Autodesk Fusion 360 part; units mm, degrees
(part 2 of 3)
  spline S100 degree 3 poles (29.5625, 4.9912) (29.775, 5.0168) (30.2128, 5.0697) (30.5239, 5.3836) (30.6839, 5.5451) knots 0 0 0 0 0.062335 0.128396 0.128396 0.128396 0.128396
  spline S101 degree 3 poles (30.6839, 5.5451) (30.8194, 5.7748) (31.1299, 6.3011) (31.1431, 6.9153) (31.1505, 7.2613) knots 0 0 0 0 0.078797 0.180491 0.180491 0.180491 0.180491
  spline S102 degree 3 poles (31.1505, 7.2613) (31.1422, 7.593) (31.1274, 8.1866) (30.8272, 8.6957) (30.6948, 8.9203) knots 0 0 0 0 0.09753 0.174557 0.174557 0.174557 0.174557
  spline S103 degree 3 poles (30.6948, 8.9203) (30.5395, 9.081) (30.2395, 9.3914) (29.8122, 9.4454) (29.6061, 9.4714) knots 0 0 0 0 0.064875 0.125334 0.125334 0.125334 0.125334
  spline S104 degree 3 poles (29.6061, 9.4714) (29.399, 9.442) (28.9607, 9.3797) (28.6562, 9.0557) (28.4956, 8.8848) knots 0 0 0 0 0.060932 0.128979 0.128979 0.128979 0.128979
  spline S105 degree 3 poles (28.4956, 8.8848) (28.3552, 8.6509) (28.0416, 8.1287) (28.023, 7.5171) (28.0127, 7.1795) knots 0 0 0 0 0.080566 0.17987 0.17987 0.17987 0.17987
  line L143 (35.4834, 5.1931) -> (35.6252, 4.3254)
  spline S106 degree 3 poles (35.6252, 4.3254) (35.4947, 4.3) (35.2494, 4.2522) (34.9998, 4.2426) (34.8831, 4.2381) knots 0 0 0 0 0.039832 0.074826 0.074826 0.074826 0.074826
  spline S107 degree 3 poles (34.8831, 4.2381) (34.7224, 4.2412) (34.4348, 4.2468) (34.1703, 4.3581) (34.0536, 4.4073) knots 0 0 0 0 0.047664 0.085336 0.085336 0.085336 0.085336
  spline S108 degree 3 poles (34.0536, 4.4073) (33.9634, 4.4665) (33.7887, 4.5812) (33.6877, 4.7638) (33.6389, 4.8521) knots 0 0 0 0 0.031834 0.061632 0.061632 0.061632 0.061632
  spline S109 degree 3 poles (33.6389, 4.8521) (33.6044, 4.9941) (33.512, 5.3741) (33.5162, 5.7661) (33.5188, 6.0117) knots 0 0 0 0 0.043707 0.116961 0.116961 0.116961 0.116961
  line L144 (33.5188, 6.0117) -> (33.5188, 9.3459)
  line L145 (33.5188, 9.3459) -> (32.7985, 9.3459)
  line L146 (32.7985, 9.3459) -> (32.7985, 10.1099)
  line L147 (32.7985, 10.1099) -> (33.5188, 10.1099)
  line L148 (33.5188, 10.1099) -> (33.5188, 11.5451)
  line L149 (33.5188, 11.5451) -> (34.4956, 12.1345)
  line L150 (34.4956, 12.1345) -> (34.4956, 10.1099)
  line L151 (34.4956, 10.1099) -> (35.4834, 10.1099)
  line L152 (35.4834, 10.1099) -> (35.4834, 9.3459)
  line L153 (35.4834, 9.3459) -> (34.4956, 9.3459)
  line L154 (34.4956, 9.3459) -> (34.4956, 5.9571)
  spline S110 degree 3 poles (34.4956, 5.9571) (34.4942, 5.8414) (34.4919, 5.659) (34.5326, 5.4817) (34.5475, 5.4169) knots 0 0 0 0 0.03454 0.054433 0.054433 0.054433 0.054433
  spline S111 degree 3 poles (34.5475, 5.4169) (34.5677, 5.3787) (34.6088, 5.3015) (34.6804, 5.2513) (34.7166, 5.2259) knots 0 0 0 0 0.012755 0.025838 0.025838 0.025838 0.025838
  spline S112 degree 3 poles (34.7166, 5.2259) (34.7635, 5.2052) (34.8701, 5.1584) (34.9868, 5.1562) (35.0522, 5.1549) knots 0 0 0 0 0.015217 0.034603 0.034603 0.034603 0.034603
  spline S113 degree 3 poles (35.0522, 5.1549) (35.1155, 5.1572) (35.2599, 5.1623) (35.403, 5.182) (35.4834, 5.1931) knots 0 0 0 0 0.018987 0.043304 0.043304 0.043304 0.043304
  line L155 (36.4001, 2.0826) -> (36.291, 3.0048)
  spline S114 degree 3 poles (36.291, 3.0048) (36.391, 2.9794) (36.5756, 2.9325) (36.7658, 2.9222) (36.8531, 2.9175) knots 0 0 0 0 0.030853 0.057001 0.057001 0.057001 0.057001
  spline S115 degree 3 poles (36.8531, 2.9175) (36.9528, 2.92) (37.1344, 2.9246) (37.3015, 2.9949) (37.3769, 3.0267) knots 0 0 0 0 0.029594 0.053932 0.053932 0.053932 0.053932
  spline S116 degree 3 poles (37.3769, 3.0267) (37.4397, 3.067) (37.5663, 3.1484) (37.6544, 3.2706) (37.6989, 3.3323) knots 0 0 0 0 0.022157 0.044743 0.044743 0.044743 0.044743
  spline S117 degree 3 poles (37.6989, 3.3323) (37.7407, 3.4172) (37.8571, 3.654) (37.9436, 3.9035) (37.999, 4.0635) knots 0 0 0 0 0.028377 0.079105 0.079105 0.079105 0.079105
  spline S118 degree 3 poles (37.999, 4.0635) (38.0107, 4.0972) (38.0387, 4.1777) (38.0688, 4.2573) (38.0864, 4.3036) knots 0 0 0 0 0.0107 0.02555 0.02555 0.02555 0.02555
  line L156 (38.0864, 4.3036) -> (35.8872, 10.1099)
  line L157 (35.8872, 10.1099) -> (36.9458, 10.1099)
  line L158 (36.9458, 10.1099) -> (38.1518, 6.7538)
  spline S119 degree 3 poles (38.1518, 6.7538) (38.2285, 6.5363) (38.3845, 6.0939) (38.5088, 5.6414) (38.572, 5.4114) knots 0 0 0 0 0.069157 0.140705 0.140705 0.140705 0.140705
  spline S120 degree 3 poles (38.572, 5.4114) (38.631, 5.6351) (38.7483, 6.0806) (38.9002, 6.5155) (38.9759, 6.732) knots 0 0 0 0 0.069376 0.138143 0.138143 0.138143 0.138143
  line L159 (38.9759, 6.732) -> (40.2146, 10.1099)
  line L160 (40.2146, 10.1099) -> (41.1969, 10.1099)
  line L161 (41.1969, 10.1099) -> (38.9922, 4.2163)
  spline S121 degree 3 poles (38.9922, 4.2163) (38.8921, 3.9454) (38.7272, 3.499) (38.5218, 3.0699) (38.4411, 2.9012) knots 0 0 0 0 0.086568 0.142661 0.142661 0.142661 0.142661
  spline S122 degree 3 poles (38.4411, 2.9012) (38.3557, 2.7537) (38.1975, 2.4803) (37.9533, 2.2809) (37.8408, 2.189) knots 0 0 0 0 0.050608 0.093822 0.093822 0.093822 0.093822
  spline S123 degree 3 poles (37.8408, 2.189) (37.7198, 2.123) (37.4683, 1.9857) (37.1818, 1.9705) (37.0332, 1.9626) knots 0 0 0 0 0.04081 0.084832 0.084832 0.084832 0.084832
  spline S124 degree 3 poles (37.0332, 1.9626) (36.9324, 1.9688) (36.7165, 1.9821) (36.5102, 2.0476) (36.4001, 2.0826) knots 0 0 0 0 0.030163 0.064648 0.064648 0.064648 0.064648
extrude "Extrude11'" cut sketch "Sketch9" against normal blind 0.1 contours L94 L95 L96 S34 S35 S36 S37 S38 S39 S40 S41 S42 S43 L97 L98 sketch seen with x (1, 0, 0) y (0, 0, -1) z (0, 1, 0) at (0, -23.4903, 46.4903) bodies 3 in component "Component"
extrude "Extrude12'" cut sketch "Sketch9" against normal blind 0.1 contours L76 L77 L78 L79 L80 L81 L82 L83 L84 L85 L86 L87 | L88 S0 S1 S2 S3 S4 S5 S6 S7 S8 L89 S9 S10 S11 S12 | L91 S17 S18 S19 S20 S21 S22 S23 S24 S25 L92 S26 S27 S28 S29 | L99 L100 L101 S52 S53 L102 L103 L104 L105 L106 L107 L108 L109 L110 L111 | L112 S54 S55 S56 S57 S58 S59 S60 S61 S62 L113 S63 S64 S65 S66 | L115 L116 L117 L118 L119 L120 L121 L122 L123 L124 L125 L126 | L127 L128 L129 S71 S72 S73 S74 S75 S76 S77 L130 L131 L132 S78 S79 S80 S81 S82 L133 L134 L135 S83 S84 S85 S86 S87 L136 L137 | L138 L139 L140 S88 S89 S90 S91 S92 S93 S94 S95 S96 S97 L141 L142 | L143 S106 S107 S108 S109 L144 L145 L146 L147 L148 L149 L150 L151 L152 L153 L154 S110 S111 S112 S113 | L155 S114 S115 S116 S117 S118 L156 L157 L158 S119 S120 L159 L160 L161 S121 S122 S123 S124 sketch seen with x (1, 0, 0) y (0, 0, -1) z (0, 1, 0) at (0, -23.4903, 46.4903) bodies 3 in component "Component"
sketch "Sketch10" plane through (0, 0, 22.6977) normal (0, 0, 1) x (1, 0, 0)
  line L0 (-6.4359, 98.3368) -> (-6.4359, 103.3368)
  line L1 (-6.4359, 103.3368) -> (-8.4359, 103.3368)
  line L2 (-8.4359, 103.3368) -> (-8.4359, 108.3368)
  line L3 (-8.4359, 108.3368) -> (-6.4359, 108.3368)
  line L4 (-6.4359, 108.3368) -> (-6.4359, 113.3368)
  line L5 (-6.4359, 113.3368) -> (-56.4359, 113.3368)
  line L6 (-56.4359, 113.3368) -> (-56.4359, 108.3368)
  line L7 (-56.4359, 108.3368) -> (-53.4359, 108.3368)
  line L8 (-53.4359, 108.3368) -> (-53.4359, 103.3368)
  line L9 (-53.4359, 103.3368) -> (-56.4359, 103.3368)
  line L10 (-56.4359, 103.3368) -> (-56.4359, 98.3368)
  line L11 (-56.4359, 98.3368) -> (-53.4359, 98.3368)
  line L12 (-53.4359, 98.3368) -> (-53.4359, 93.3368)
  line L13 (-53.4359, 93.3368) -> (-56.4359, 93.3368)
  line L14 (-56.4359, 93.3368) -> (-56.4359, 88.3368)
  line L15 (-56.4359, 88.3368) -> (-53.4359, 88.3368)
  line L16 (-53.4359, 88.3368) -> (-53.4359, 83.3368)
  line L17 (-53.4359, 83.3368) -> (-56.4359, 83.3368)
  line L18 (-56.4359, 83.3368) -> (-56.4359, 78.3368)
  line L19 (-56.4359, 78.3368) -> (-53.4359, 78.3368)
  line L20 (-53.4359, 78.3368) -> (-53.4359, 73.3368)
  line L21 (-53.4359, 73.3368) -> (-56.4359, 73.3368)
  line L22 (-56.4359, 73.3368) -> (-56.4359, 68.3368)
  line L23 (-56.4359, 68.3368) -> (-46.7359, 68.3368)
  line L24 (-46.7359, 68.3368) -> (-46.7359, 65.8368)
  line L25 (-46.7359, 65.8368) -> (-41.3359, 65.8368)
  line L26 (-41.3359, 65.8368) -> (-41.3359, 68.3368)
  line L27 (-41.3359, 68.3368) -> (-36.7359, 68.3368)
  line L28 (-36.7359, 68.3368) -> (-36.7359, 65.8368)
  line L29 (-36.7359, 65.8368) -> (-31.3359, 65.8368)
  line L30 (-31.3359, 65.8368) -> (-31.3359, 68.3368)
  line L31 (-31.3359, 68.3368) -> (-26.7359, 68.3368)
  line L32 (-26.7359, 68.3368) -> (-26.7359, 65.8368)
  line L33 (-26.7359, 65.8368) -> (-21.3359, 65.8368)
  line L34 (-21.3359, 65.8368) -> (-21.3359, 68.3368)
  line L35 (-21.3359, 68.3368) -> (-16.7359, 68.3368)
  line L36 (-16.7359, 68.3368) -> (-16.7359, 65.8368)
  line L37 (-16.7359, 65.8368) -> (-11.3359, 65.8368)
  line L38 (-11.3359, 65.8368) -> (-11.3359, 68.3368)
  line L39 (-11.3359, 68.3368) -> (-6.4359, 68.3368)
  line L40 (-6.4359, 68.3368) -> (-6.4359, 73.3368)
  line L41 (-6.4359, 73.3368) -> (-8.4359, 73.3368)
  line L42 (-8.4359, 73.3368) -> (-8.4359, 78.3368)
  line L43 (-8.4359, 78.3368) -> (-6.4359, 78.3368)
  line L44 (-6.4359, 78.3368) -> (-6.4359, 83.3368)
  line L45 (-6.4359, 83.3368) -> (-8.4359, 83.3368)
  line L46 (-8.4359, 83.3368) -> (-8.4359, 88.3368)
  line L47 (-8.4359, 88.3368) -> (-6.4359, 88.3368)
  line L48 (-6.4359, 88.3368) -> (-6.4359, 93.3368)
  line L49 (-6.4359, 93.3368) -> (-8.4359, 93.3368)
  line L50 (-8.4359, 93.3368) -> (-8.4359, 98.3368)
  line L51 (-8.4359, 98.3368) -> (-6.4359, 98.3368)
  line L52 (-44.847, 105.1125) -> (-15.0997, 105.1125)
  line L53 (-15.0997, 105.1125) -> (-15.0997, 75.3652)
  line L54 (-15.0997, 75.3652) -> (-44.847, 75.3652)
  line L55 (-44.847, 75.3652) -> (-44.847, 105.1125)
  line L56 (-44.847, 105.1125) -> (-15.0997, 105.1125)
  line L57 (-44.847, 75.3652) -> (-44.847, 105.1125)
  line L58 (-15.0997, 75.3652) -> (-44.847, 75.3652)
  line L59 (-15.0997, 105.1125) -> (-15.0997, 75.3652)
  line L60 (-29.9733, 105.1125) -> (-29.9733, 75.3652) construction
  line L61 (-44.847, 90.2388) -> (-15.0997, 90.2388) construction
  line L62 (-8.6718, 90.2601) -> (-29.7064, 69.2256)
  line L63 (-29.7064, 69.2256) -> (-50.7409, 90.2601)
  line L64 (-29.7064, 111.2947) -> (-8.6718, 90.2601)
  line L65 (-50.7409, 90.2601) -> (-29.7064, 111.2947)
  line L66 (-16.0997, 76.3652) -> (-43.847, 76.3652)
  line L67 (-43.847, 76.3652) -> (-43.847, 104.1125)
  line L68 (-43.847, 104.1125) -> (-16.0997, 104.1125)
  line L69 (-16.0997, 104.1125) -> (-16.0997, 76.3652)
  line L70 (-49.3267, 90.2601) -> (-29.7064, 109.8804)
  line L71 (-29.7064, 109.8804) -> (-10.086, 90.2601)
  line L72 (-10.086, 90.2601) -> (-29.7064, 70.6398)
  line L73 (-29.7064, 70.6398) -> (-49.3267, 90.2601)
  dimension "d133" = 1
  dimension "d134" = 1
  constraint horizontal L52
  constraint vertical L53
  constraint horizontal L54
  constraint vertical L55
  constraint horizontal L56
  constraint vertical L59
  constraint horizontal L58
  constraint vertical L57
  constraint midpoint L56 L60.start
  constraint midpoint L54 L60.end
  constraint perpendicular L54 L60
  constraint midpoint L57 L61.start
  constraint midpoint L59 L61.end
extrude "Extrude3''" cut sketch "Sketch10" against normal blind 3 contours L52 L56 L70 L71 | L65 L67 L68 | L55 L57 L70 L73 | L66 L67 L68 L69 L70 L71 L72 L73 | L64 L68 L69 | L63 L66 L67 | L53 L59 L71 L72 | L54 L58 L72 L73 | L62 L66 L69 sketch seen with x (0, 0, -1) y (0, 1, 0) z (1, 0, 0) at (-19.6977, -54.1484, -8.993) bodies 4 in component "Component''"
sketch "Sketch11" plane through (0, 0, 2.5) normal (0, 0, 1) x (1, 0, 0)
  line L0 (47.5, 60) -> (47.5, 67.3)
  line L1 (47.5, 67.3) -> (50, 67.3)
  line L2 (50, 67.3) -> (50, 72.7)
  line L3 (50, 72.7) -> (47.5, 72.7)
  line L4 (47.5, 72.7) -> (47.5, 77.3)
  line L5 (47.5, 77.3) -> (50, 77.3)
  line L6 (50, 77.3) -> (50, 82.7)
  line L7 (50, 82.7) -> (47.5, 82.7)
  line L8 (47.5, 82.7) -> (47.5, 87.3)
  line L9 (47.5, 87.3) -> (50, 87.3)
  line L10 (50, 87.3) -> (50, 92.7)
  line L11 (50, 92.7) -> (47.5, 92.7)
  line L12 (47.5, 92.7) -> (47.5, 97.3)
  line L13 (47.5, 97.3) -> (50, 97.3)
  line L14 (50, 97.3) -> (50, 102.7)
  line L15 (50, 102.7) -> (47.5, 102.7)
  line L16 (47.5, 102.7) -> (47.5, 107.5)
  line L17 (47.5, 107.5) -> (2.5, 107.5)
  line L18 (2.5, 107.5) -> (2.5, 102.7)
  line L19 (2.5, 102.7) -> (0, 102.7)
  line L20 (0, 102.7) -> (0, 97.3)
  line L21 (0, 97.3) -> (2.5, 97.3)
  line L22 (2.5, 97.3) -> (2.5, 92.7)
  line L23 (2.5, 92.7) -> (0, 92.7)
  line L24 (0, 92.7) -> (0, 87.3)
  line L25 (0, 87.3) -> (2.5, 87.3)
  line L26 (2.5, 87.3) -> (2.5, 82.7)
  line L27 (2.5, 82.7) -> (0, 82.7)
  line L28 (0, 82.7) -> (0, 77.3)
  line L29 (0, 77.3) -> (2.5, 77.3)
  line L30 (2.5, 77.3) -> (2.5, 72.7)
  line L31 (2.5, 72.7) -> (0, 72.7)
  line L32 (0, 72.7) -> (0, 67.3)
  line L33 (0, 67.3) -> (2.5, 67.3)
  line L34 (2.5, 67.3) -> (2.5, 60)
  line L35 (2.5, 60) -> (7.5, 60)
  line L36 (7.5, 60) -> (7.5, 63)
  line L37 (7.5, 63) -> (12.5, 63)
  line L38 (12.5, 63) -> (12.5, 60)
  line L39 (12.5, 60) -> (17.5, 60)
  line L40 (17.5, 60) -> (17.5, 63)
  line L41 (17.5, 63) -> (22.5, 63)
  line L42 (22.5, 63) -> (22.5, 60)
  line L43 (22.5, 60) -> (27.5, 60)
  line L44 (27.5, 60) -> (27.5, 63)
  line L45 (27.5, 63) -> (32.5, 63)
  line L46 (32.5, 63) -> (32.5, 60)
  line L47 (32.5, 60) -> (37.5, 60)
  line L48 (37.5, 60) -> (37.5, 63)
  line L49 (37.5, 63) -> (42.5, 63)
  line L50 (42.5, 63) -> (42.5, 60)
  line L51 (42.5, 60) -> (47.5, 60)
  circle A0 centre (24.774, 85.3016) radius 17.2854
  circle A1 centre (24.774, 85.3016) radius 15.2854
  circle A2 centre (24.774, 85.3016) radius 13.2854
  circle A3 centre (24.774, 85.3016) radius 11.2854
  circle A4 centre (24.774, 85.3016) radius 9.2854
  line L52 (24.774, 85.3016) -> (24.774, 102.587)
  line L53 (24.774, 85.3016) -> (24.774, 68.0163)
  line L54 (24.774, 85.3016) -> (30.1155, 68.8623)
  line L55 (24.774, 85.3016) -> (19.4325, 101.741)
  line L56 (24.774, 85.3016) -> (34.9341, 71.3175)
  line L57 (24.774, 85.3016) -> (14.6139, 99.2858)
  line L58 (24.774, 85.3016) -> (38.7582, 75.1416)
  line L59 (24.774, 85.3016) -> (10.7899, 95.4617)
  line L60 (24.774, 85.3016) -> (41.2134, 79.9602)
  line L61 (24.774, 85.3016) -> (8.3347, 90.6431)
  line L62 (24.774, 85.3016) -> (42.0594, 85.3016)
  line L63 (24.774, 85.3016) -> (7.4886, 85.3016)
  line L64 (24.774, 85.3016) -> (41.2134, 90.6431)
  line L65 (24.774, 85.3016) -> (8.3347, 79.9602)
  line L66 (24.774, 85.3016) -> (38.7582, 95.4617)
  line L67 (24.774, 85.3016) -> (10.7899, 75.1416)
  line L68 (24.774, 85.3016) -> (34.9341, 99.2858)
  line L69 (24.774, 85.3016) -> (14.6139, 71.3175)
  line L70 (24.774, 85.3016) -> (30.1155, 101.741)
  line L71 (24.774, 85.3016) -> (19.4325, 68.8623)
  line L72 (24.774, 85.3016) -> (24.774, 102.587)
  line L73 (24.774, 85.3016) -> (24.774, 68.0163)
  line L74 (24.774, 85.3016) -> (19.4325, 101.741)
  line L75 (24.774, 85.3016) -> (30.1155, 68.8623)
  line L76 (24.774, 85.3016) -> (14.6139, 99.2858)
  line L77 (24.774, 85.3016) -> (34.9341, 71.3175)
  line L78 (24.774, 85.3016) -> (10.7899, 95.4617)
  line L79 (24.774, 85.3016) -> (38.7582, 75.1416)
  line L80 (24.774, 85.3016) -> (8.3347, 90.6431)
  line L81 (24.774, 85.3016) -> (41.2134, 79.9602)
  line L82 (24.774, 85.3016) -> (7.4886, 85.3016)
  line L83 (24.774, 85.3016) -> (42.0594, 85.3016)
  line L84 (24.774, 85.3016) -> (8.3347, 79.9602)
  line L85 (24.774, 85.3016) -> (41.2134, 90.6431)
  line L86 (24.774, 85.3016) -> (10.7899, 75.1416)
  line L87 (24.774, 85.3016) -> (38.7582, 95.4617)
  line L88 (24.774, 85.3016) -> (14.6139, 71.3175)
  line L89 (24.774, 85.3016) -> (34.9341, 99.2858)
  line L90 (24.774, 85.3016) -> (19.4325, 68.8623)
  line L91 (24.774, 85.3016) -> (30.1155, 101.741)
  dimension "d137" = -2
  dimension "d138" = -4
  dimension "d139" = -6
  dimension "d140" = -8
  dimension "d142" = 360
  constraint coincident A0.centre A1.centre
  constraint coincident A0 L52.end
  constraint vertical L52
  constraint coincident A0 L53.end
  constraint parallel L52 L53
extrude "Extrude1'''" cut sketch "Sketch11" against normal blind 3 contours A0 A1 L62 L64 L83 L85 | A0 A1 L58 L60 L79 L81 | A0 A1 L66 L68 L87 L89 | A2 A3 L62 L64 L83 L85 | A0 A1 L54 L56 L75 L77 | A2 A3 L58 L60 L79 L81 | A0 A1 L52 L70 L72 L91 | A2 A3 L66 L68 L87 L89 | A4 L62 L64 L83 L85 | A0 A1 L53 L71 L73 L90 | A2 A3 L54 L56 L75 L77 | A4 L58 L60 L79 L81 | A4 L54 L56 L75 L77 | A4 L55 L57 L74 L76 | A4 L59 L61 L78 L80 | A4 L63 L65 L82 L84 | A4 L66 L68 L87 L89 | A4 L67 L69 L86 L88 | A4 L52 L70 L72 L91 | A4 L53 L71 L73 L90 | A0 A1 L55 L57 L74 L76 | A2 A3 L52 L70 L72 L91 | A0 A1 L67 L69 L86 L88 | A2 A3 L53 L71 L73 L90 | A2 A3 L55 L57 L74 L76 | A2 A3 L59 L61 L78 L80 | A2 A3 L63 L65 L82 L84 | A2 A3 L67 L69 L86 L88 | A0 A1 L59 L61 L78 L80 | A0 A1 L63 L65 L82 L84 sketch seen with x (1, 0, 0) y (0, 1, 0) z (0, 0, 1) at (0, -60, -2.5) bodies 6 in component "Component'''"
sketch "Sketch13" plane through (0, 0, 22.6977) normal (0, 0, 1) x (1, 0, 0)
  line L0 (-29.7064, 70.6398) -> (-34.4317, 75.3652)
  line L1 (-34.4317, 75.3652) -> (-24.981, 75.3652)
  line L2 (-24.981, 75.3652) -> (-29.7064, 70.6398)
  line L3 (-29.7064, 109.8804) -> (-24.9384, 105.1125)
  line L4 (-24.9384, 105.1125) -> (-34.4743, 105.1125)
  line L5 (-34.4743, 105.1125) -> (-29.7064, 109.8804)
  line L6 (-43.847, 104.1125) -> (-36.8885, 104.1125)
  line L7 (-36.8885, 104.1125) -> (-43.847, 97.154)
  line L8 (-43.847, 97.154) -> (-43.847, 104.1125)
  line L9 (-22.5668, 76.3652) -> (-16.0997, 82.8323)
  line L10 (-16.0997, 82.8323) -> (-16.0997, 76.3652)
  line L11 (-16.0997, 76.3652) -> (-22.5668, 76.3652)
  line L12 (-43.847, 76.3652) -> (-43.847, 83.3662)
  line L13 (-43.847, 83.3662) -> (-36.8459, 76.3652)
  line L14 (-36.8459, 76.3652) -> (-43.847, 76.3652)
  line L15 (-16.0997, 104.1125) -> (-16.0997, 97.688)
  line L16 (-16.0997, 97.688) -> (-22.5242, 104.1125)
  line L17 (-22.5242, 104.1125) -> (-16.0997, 104.1125)
  line L18 (-16.0997, 96.2738) -> (-16.0997, 84.2465)
  line L19 (-16.0997, 84.2465) -> (-23.981, 76.3652)
  line L20 (-23.981, 76.3652) -> (-35.4317, 76.3652)
  line L21 (-35.4317, 76.3652) -> (-43.847, 84.7805)
  line L22 (-43.847, 84.7805) -> (-43.847, 95.7398)
  line L23 (-43.847, 95.7398) -> (-35.4743, 104.1125)
  line L24 (-35.4743, 104.1125) -> (-23.9384, 104.1125)
  line L25 (-23.9384, 104.1125) -> (-16.0997, 96.2738)
  line L26 (-10.086, 90.2601) -> (-15.0997, 85.2465)
  line L27 (-15.0997, 85.2465) -> (-15.0997, 95.2738)
  line L28 (-15.0997, 95.2738) -> (-10.086, 90.2601)
  line L29 (-44.847, 94.7398) -> (-44.847, 85.7805)
  line L30 (-44.847, 85.7805) -> (-49.3267, 90.2601)
  line L31 (-49.3267, 90.2601) -> (-44.847, 94.7398)
  line L32 (-6.4359, 98.3368) -> (-6.4359, 103.3368)
  line L33 (-6.4359, 103.3368) -> (-8.4359, 103.3368)
  line L34 (-8.4359, 103.3368) -> (-8.4359, 108.3368)
  line L35 (-8.4359, 108.3368) -> (-6.4359, 108.3368)
  line L36 (-6.4359, 108.3368) -> (-6.4359, 113.3368)
  line L37 (-6.4359, 113.3368) -> (-56.4359, 113.3368)
  line L38 (-56.4359, 113.3368) -> (-56.4359, 108.3368)
  line L39 (-56.4359, 108.3368) -> (-53.4359, 108.3368)
  line L40 (-53.4359, 108.3368) -> (-53.4359, 103.3368)
  line L41 (-53.4359, 103.3368) -> (-56.4359, 103.3368)
  line L42 (-56.4359, 103.3368) -> (-56.4359, 98.3368)
  line L43 (-56.4359, 98.3368) -> (-53.4359, 98.3368)
  line L44 (-53.4359, 98.3368) -> (-53.4359, 93.3368)
  line L45 (-53.4359, 93.3368) -> (-56.4359, 93.3368)
  line L46 (-56.4359, 93.3368) -> (-56.4359, 88.3368)
  line L47 (-56.4359, 88.3368) -> (-53.4359, 88.3368)
  line L48 (-53.4359, 88.3368) -> (-53.4359, 83.3368)
  line L49 (-53.4359, 83.3368) -> (-56.4359, 83.3368)
  line L50 (-56.4359, 83.3368) -> (-56.4359, 78.3368)
  line L51 (-56.4359, 78.3368) -> (-53.4359, 78.3368)
  line L52 (-53.4359, 78.3368) -> (-53.4359, 73.3368)
  line L53 (-53.4359, 73.3368) -> (-56.4359, 73.3368)
  line L54 (-56.4359, 73.3368) -> (-56.4359, 68.3368)
  line L55 (-56.4359, 68.3368) -> (-46.7359, 68.3368)
  line L56 (-46.7359, 68.3368) -> (-46.7359, 65.8368)
  line L57 (-46.7359, 65.8368) -> (-41.3359, 65.8368)
  line L58 (-41.3359, 65.8368) -> (-41.3359, 68.3368)
  line L59 (-41.3359, 68.3368) -> (-36.7359, 68.3368)
  line L60 (-36.7359, 68.3368) -> (-36.7359, 65.8368)
  line L61 (-36.7359, 65.8368) -> (-31.3359, 65.8368)
  line L62 (-31.3359, 65.8368) -> (-31.3359, 68.3368)
  line L63 (-31.3359, 68.3368) -> (-26.7359, 68.3368)
  line L64 (-26.7359, 68.3368) -> (-26.7359, 65.8368)
  line L65 (-26.7359, 65.8368) -> (-21.3359, 65.8368)
  line L66 (-21.3359, 65.8368) -> (-21.3359, 68.3368)
  line L67 (-21.3359, 68.3368) -> (-16.7359, 68.3368)
  line L68 (-16.7359, 68.3368) -> (-16.7359, 65.8368)
  line L69 (-16.7359, 65.8368) -> (-11.3359, 65.8368)
  line L70 (-11.3359, 65.8368) -> (-11.3359, 68.3368)
  line L71 (-11.3359, 68.3368) -> (-6.4359, 68.3368)
  line L72 (-6.4359, 68.3368) -> (-6.4359, 73.3368)
  line L73 (-6.4359, 73.3368) -> (-8.4359, 73.3368)
  line L74 (-8.4359, 73.3368) -> (-8.4359, 78.3368)
  line L75 (-8.4359, 78.3368) -> (-6.4359, 78.3368)
  line L76 (-6.4359, 78.3368) -> (-6.4359, 83.3368)
  line L77 (-6.4359, 83.3368) -> (-8.4359, 83.3368)
  line L78 (-8.4359, 83.3368) -> (-8.4359, 88.3368)
  line L79 (-8.4359, 88.3368) -> (-6.4359, 88.3368)
  line L80 (-6.4359, 88.3368) -> (-6.4359, 93.3368)
  line L81 (-6.4359, 93.3368) -> (-8.4359, 93.3368)
  line L82 (-8.4359, 93.3368) -> (-8.4359, 98.3368)
  line L83 (-8.4359, 98.3368) -> (-6.4359, 98.3368)
  line L84 (31.4074, 94.4317) -> (32.5829, 96.0497)
  arc A0 (35.5221, 93.1106) -> (32.5829, 96.0497) centre (24.774, 85.3016) ccw
  line L85 (35.5221, 93.1106) -> (33.9041, 91.935)
  arc A1 (33.9041, 91.935) -> (31.4074, 94.4317) centre (24.774, 85.3016) ccw
  line L86 (35.507, 81.8143) -> (37.4091, 81.1962)
  arc A2 (35.5221, 77.4927) -> (37.4091, 81.1962) centre (24.774, 85.3016) ccw
  line L87 (35.5221, 77.4927) -> (33.9041, 78.6683)
  arc A3 (33.9041, 78.6683) -> (35.507, 81.8143) centre (24.774, 85.3016) ccw
  arc A4 (20.6686, 72.6665) -> (24.774, 72.0163) centre (24.774, 85.3016) ccw
  line L88 (20.6686, 72.6665) -> (21.2866, 74.5686)
  arc A5 (21.2866, 74.5686) -> (24.774, 74.0163) centre (24.774, 85.3016) ccw
  line L89 (24.774, 74.0163) -> (24.774, 72.0163)
  line L90 (14.041, 81.8143) -> (12.1389, 81.1962)
  arc A6 (11.4886, 85.3016) -> (12.1389, 81.1962) centre (24.774, 85.3016) ccw
  line L91 (11.4886, 85.3016) -> (13.4886, 85.3016)
  arc A7 (13.4886, 85.3016) -> (14.041, 81.8143) centre (24.774, 85.3016) ccw
  line L92 (18.1406, 94.4317) -> (16.9651, 96.0497)
  arc A8 (20.6686, 97.9368) -> (16.9651, 96.0497) centre (24.774, 85.3016) ccw
  line L93 (20.6686, 97.9368) -> (21.2866, 96.0347)
  arc A9 (21.2866, 96.0347) -> (18.1406, 94.4317) centre (24.774, 85.3016) ccw
  line L94 (14.041, 88.789) -> (12.1389, 89.407)
  arc A10 (14.0259, 93.1106) -> (12.1389, 89.407) centre (24.774, 85.3016) ccw
  line L95 (14.0259, 93.1106) -> (15.644, 91.935)
  arc A11 (15.644, 91.935) -> (14.041, 88.789) centre (24.774, 85.3016) ccw
  line L96 (18.1406, 76.1716) -> (16.9651, 74.5536)
  arc A12 (14.0259, 77.4927) -> (16.9651, 74.5536) centre (24.774, 85.3016) ccw
  line L97 (14.0259, 77.4927) -> (15.644, 78.6683)
  arc A13 (15.644, 78.6683) -> (18.1406, 76.1716) centre (24.774, 85.3016) ccw
  line L98 (31.4074, 76.1716) -> (32.5829, 74.5536)
  arc A14 (28.8794, 72.6665) -> (32.5829, 74.5536) centre (24.774, 85.3016) ccw
  line L99 (28.8794, 72.6665) -> (28.2614, 74.5686)
  arc A15 (28.2614, 74.5686) -> (31.4074, 76.1716) centre (24.774, 85.3016) ccw
  line L100 (35.507, 88.789) -> (37.4091, 89.407)
  arc A16 (38.0594, 85.3016) -> (37.4091, 89.407) centre (24.774, 85.3016) ccw
  line L101 (38.0594, 85.3016) -> (36.0594, 85.3016)
  arc A17 (36.0594, 85.3016) -> (35.507, 88.789) centre (24.774, 85.3016) ccw
  arc A18 (28.8794, 97.9368) -> (24.774, 98.587) centre (24.774, 85.3016) ccw
  line L102 (28.8794, 97.9368) -> (28.2614, 96.0347)
  arc A19 (28.2614, 96.0347) -> (24.774, 96.587) centre (24.774, 85.3016) ccw
  line L103 (24.774, 96.587) -> (24.774, 98.587)
  line L104 (33.7585, 97.6678) -> (34.9341, 99.2858)
  arc A20 (38.7582, 95.4617) -> (34.9341, 99.2858) centre (24.774, 85.3016) ccw
  line L105 (38.7582, 95.4617) -> (37.1401, 94.2862)
  arc A21 (37.1401, 94.2862) -> (33.7585, 97.6678) centre (24.774, 85.3016) ccw
  line L106 (39.3112, 80.5782) -> (41.2134, 79.9602)
  arc A22 (38.7582, 75.1416) -> (41.2134, 79.9602) centre (24.774, 85.3016) ccw
  line L107 (38.7582, 75.1416) -> (37.1401, 76.3171)
  arc A23 (37.1401, 76.3171) -> (39.3112, 80.5782) centre (24.774, 85.3016) ccw
  arc A24 (19.4325, 68.8623) -> (24.774, 68.0163) centre (24.774, 85.3016) ccw
  line L108 (19.4325, 68.8623) -> (20.0506, 70.7644)
  arc A25 (20.0506, 70.7644) -> (24.774, 70.0163) centre (24.774, 85.3016) ccw
  line L109 (24.774, 70.0163) -> (24.774, 68.0163)
  line L110 (10.2368, 80.5782) -> (8.3347, 79.9602)
  arc A26 (7.4886, 85.3016) -> (8.3347, 79.9602) centre (24.774, 85.3016) ccw
  line L111 (7.4886, 85.3016) -> (9.4886, 85.3016)
  arc A27 (9.4886, 85.3016) -> (10.2368, 80.5782) centre (24.774, 85.3016) ccw
  arc A28 (27.6433, 94.1325) -> (24.774, 94.587) centre (24.774, 85.3016) ccw
  line L112 (27.6433, 94.1325) -> (24.774, 85.3016)
  line L113 (24.774, 85.3016) -> (30.2318, 92.8137)
  arc A29 (32.286, 90.7594) -> (30.2318, 92.8137) centre (24.774, 85.3016) ccw
  line L114 (32.286, 90.7594) -> (24.774, 85.3016)
  line L115 (24.774, 85.3016) -> (33.6049, 88.171)
  arc A30 (34.0594, 85.3016) -> (33.6049, 88.171) centre (24.774, 85.3016) ccw
  line L116 (34.0594, 85.3016) -> (24.774, 85.3016)
  line L117 (24.774, 85.3016) -> (33.6049, 82.4323)
  arc A31 (32.286, 79.8438) -> (33.6049, 82.4323) centre (24.774, 85.3016) ccw
  line L118 (32.286, 79.8438) -> (24.774, 85.3016)
  line L119 (24.774, 85.3016) -> (30.2318, 77.7896)
  arc A32 (27.6433, 76.4707) -> (30.2318, 77.7896) centre (24.774, 85.3016) ccw
  line L120 (27.6433, 76.4707) -> (24.774, 85.3016)
  line L121 (24.774, 85.3016) -> (24.774, 76.0163)
  arc A33 (21.9047, 76.4707) -> (24.774, 76.0163) centre (24.774, 85.3016) ccw
  line L122 (21.9047, 76.4707) -> (24.774, 85.3016)
  line L123 (24.774, 85.3016) -> (19.3162, 77.7896)
  arc A34 (17.262, 79.8438) -> (19.3162, 77.7896) centre (24.774, 85.3016) ccw
  line L124 (17.262, 79.8438) -> (24.774, 85.3016)
  line L125 (24.774, 85.3016) -> (15.9431, 82.4323)
  arc A35 (15.4886, 85.3016) -> (15.9431, 82.4323) centre (24.774, 85.3016) ccw
  line L126 (15.4886, 85.3016) -> (24.774, 85.3016)
  line L127 (24.774, 85.3016) -> (15.9431, 88.171)
  arc A36 (17.262, 90.7594) -> (15.9431, 88.171) centre (24.774, 85.3016) ccw
  line L128 (17.262, 90.7594) -> (24.774, 85.3016)
  line L129 (24.774, 85.3016) -> (19.3162, 92.8137)
  arc A37 (21.9047, 94.1325) -> (19.3162, 92.8137) centre (24.774, 85.3016) ccw
  line L130 (21.9047, 94.1325) -> (24.774, 85.3016)
  line L131 (24.774, 85.3016) -> (24.774, 94.587)
  line L132 (15.7895, 97.6678) -> (14.6139, 99.2858)
  arc A38 (19.4325, 101.741) -> (14.6139, 99.2858) centre (24.774, 85.3016) ccw
  line L133 (19.4325, 101.741) -> (20.0506, 99.8389)
  arc A39 (20.0506, 99.8389) -> (15.7895, 97.6678) centre (24.774, 85.3016) ccw
  line L134 (10.2368, 90.0251) -> (8.3347, 90.6431)
  arc A40 (10.7899, 95.4617) -> (8.3347, 90.6431) centre (24.774, 85.3016) ccw
  line L135 (10.7899, 95.4617) -> (12.4079, 94.2862)
  arc A41 (12.4079, 94.2862) -> (10.2368, 90.0251) centre (24.774, 85.3016) ccw
  line L136 (15.7895, 72.9355) -> (14.6139, 71.3175)
  arc A42 (10.7899, 75.1416) -> (14.6139, 71.3175) centre (24.774, 85.3016) ccw
  line L137 (10.7899, 75.1416) -> (12.4079, 76.3171)
  arc A43 (12.4079, 76.3171) -> (15.7895, 72.9355) centre (24.774, 85.3016) ccw
  line L138 (33.7585, 72.9355) -> (34.9341, 71.3175)
  arc A44 (30.1155, 68.8623) -> (34.9341, 71.3175) centre (24.774, 85.3016) ccw
  line L139 (30.1155, 68.8623) -> (29.4974, 70.7644)
  arc A45 (29.4974, 70.7644) -> (33.7585, 72.9355) centre (24.774, 85.3016) ccw
  line L140 (39.3112, 90.0251) -> (41.2134, 90.6431)
  arc A46 (42.0594, 85.3016) -> (41.2134, 90.6431) centre (24.774, 85.3016) ccw
  line L141 (42.0594, 85.3016) -> (40.0594, 85.3016)
  arc A47 (40.0594, 85.3016) -> (39.3112, 90.0251) centre (24.774, 85.3016) ccw
  arc A48 (30.1155, 101.741) -> (24.774, 102.587) centre (24.774, 85.3016) ccw
  line L142 (30.1155, 101.741) -> (29.4974, 99.8389)
  arc A49 (29.4974, 99.8389) -> (24.774, 100.587) centre (24.774, 85.3016) ccw
  line L143 (24.774, 100.587) -> (24.774, 102.587)
  line L144 (47.5, 60) -> (47.5, 67.3)
  line L145 (47.5, 67.3) -> (50, 67.3)
  line L146 (50, 67.3) -> (50, 72.7)
  line L147 (50, 72.7) -> (47.5, 72.7)
  line L148 (47.5, 72.7) -> (47.5, 77.3)
  line L149 (47.5, 77.3) -> (50, 77.3)
  line L150 (50, 77.3) -> (50, 82.7)
  line L151 (50, 82.7) -> (47.5, 82.7)
  line L152 (47.5, 82.7) -> (47.5, 87.3)
  line L153 (47.5, 87.3) -> (50, 87.3)
  line L154 (50, 87.3) -> (50, 92.7)
  line L155 (50, 92.7) -> (47.5, 92.7)
  line L156 (47.5, 92.7) -> (47.5, 97.3)
  line L157 (47.5, 97.3) -> (50, 97.3)
  line L158 (50, 97.3) -> (50, 102.7)
  line L159 (50, 102.7) -> (47.5, 102.7)
  line L160 (47.5, 102.7) -> (47.5, 107.5)
  line L161 (47.5, 107.5) -> (2.5, 107.5)
  line L162 (2.5, 107.5) -> (2.5, 102.7)
  line L163 (2.5, 102.7) -> (0, 102.7)
  line L164 (0, 102.7) -> (0, 97.3)
  line L165 (0, 97.3) -> (2.5, 97.3)
  line L166 (2.5, 97.3) -> (2.5, 92.7)
  line L167 (2.5, 92.7) -> (0, 92.7)
  line L168 (0, 92.7) -> (0, 87.3)
  line L169 (0, 87.3) -> (2.5, 87.3)
  line L170 (2.5, 87.3) -> (2.5, 82.7)
  line L171 (2.5, 82.7) -> (0, 82.7)
  line L172 (0, 82.7) -> (0, 77.3)
  line L173 (0, 77.3) -> (2.5, 77.3)
  line L174 (2.5, 77.3) -> (2.5, 72.7)
  line L175 (2.5, 72.7) -> (0, 72.7)
  line L176 (0, 72.7) -> (0, 67.3)
  line L177 (0, 67.3) -> (2.5, 67.3)
  line L178 (2.5, 67.3) -> (2.5, 60)
  line L179 (2.5, 60) -> (7.5, 60)
  line L180 (7.5, 60) -> (7.5, 63)
  line L181 (7.5, 63) -> (12.5, 63)
  line L182 (12.5, 63) -> (12.5, 60)
  line L183 (12.5, 60) -> (17.5, 60)
  line L184 (17.5, 60) -> (17.5, 63)
  line L185 (17.5, 63) -> (22.5, 63)
  line L186 (22.5, 63) -> (22.5, 60)
  line L187 (22.5, 60) -> (27.5, 60)
  line L188 (27.5, 60) -> (27.5, 63)
  line L189 (27.5, 63) -> (32.5, 63)
  line L190 (32.5, 63) -> (32.5, 60)
  line L191 (32.5, 60) -> (37.5, 60)
  line L192 (37.5, 60) -> (37.5, 63)
  line L193 (37.5, 63) -> (42.5, 63)
  line L194 (42.5, 63) -> (42.5, 60)
  line L195 (42.5, 60) -> (47.5, 60)
  line L196 (94.1554, 69.5283) -> (89.4301, 64.803)
  line L197 (89.4301, 64.803) -> (84.7047, 69.5283)
  line L198 (84.7047, 69.5283) -> (94.1554, 69.5283)
  line L199 (84.6621, 99.2757) -> (89.4301, 104.0436)
  line L200 (89.4301, 104.0436) -> (94.198, 99.2757)
  line L201 (94.198, 99.2757) -> (84.6621, 99.2757)
  line L202 (96.6123, 98.2757) -> (103.5707, 98.2757)
  line L203 (103.5707, 98.2757) -> (103.5707, 91.3172)
  line L204 (103.5707, 91.3172) -> (96.6123, 98.2757)
  line L205 (75.8234, 76.9954) -> (82.2905, 70.5283)
  line L206 (82.2905, 70.5283) -> (75.8234, 70.5283)
  line L207 (75.8234, 70.5283) -> (75.8234, 76.9954)
  line L208 (103.5707, 77.5294) -> (103.5707, 70.5283)
  line L209 (103.5707, 70.5283) -> (96.5697, 70.5283)
  line L210 (96.5697, 70.5283) -> (103.5707, 77.5294)
  line L211 (75.8234, 91.8512) -> (75.8234, 98.2757)
  line L212 (75.8234, 98.2757) -> (82.2479, 98.2757)
  line L213 (82.2479, 98.2757) -> (75.8234, 91.8512)
  line L214 (75.8234, 78.4097) -> (75.8234, 90.437)
  line L215 (75.8234, 90.437) -> (83.6621, 98.2757)
  line L216 (83.6621, 98.2757) -> (95.198, 98.2757)
  line L217 (95.198, 98.2757) -> (103.5707, 89.903)
  line L218 (103.5707, 89.903) -> (103.5707, 78.9436)
  line L219 (103.5707, 78.9436) -> (95.1554, 70.5283)
  line L220 (95.1554, 70.5283) -> (83.7047, 70.5283)
  line L221 (83.7047, 70.5283) -> (75.8234, 78.4097)
  line L222 (74.8234, 79.4097) -> (69.8098, 84.4233)
  line L223 (69.8098, 84.4233) -> (74.8234, 89.437)
  line L224 (74.8234, 89.437) -> (74.8234, 79.4097)
  line L225 (104.5707, 79.9436) -> (104.5707, 88.903)
  line L226 (104.5707, 88.903) -> (109.0504, 84.4233)
  line L227 (109.0504, 84.4233) -> (104.5707, 79.9436)
  line L228 (66.1596, 97.5) -> (66.1596, 92.5)
  line L229 (66.1596, 92.5) -> (68.1596, 92.5)
  line L230 (68.1596, 92.5) -> (68.1596, 87.5)
  line L231 (68.1596, 87.5) -> (66.1596, 87.5)
  line L232 (66.1596, 87.5) -> (66.1596, 82.5)
  line L233 (66.1596, 82.5) -> (68.1596, 82.5)
  line L234 (68.1596, 82.5) -> (68.1596, 77.5)
  line L235 (68.1596, 77.5) -> (66.1596, 77.5)
  line L236 (66.1596, 77.5) -> (66.1596, 72.5)
  line L237 (66.1596, 72.5) -> (68.1596, 72.5)
  line L238 (68.1596, 72.5) -> (68.1596, 67.5)
  line L239 (68.1596, 67.5) -> (66.1596, 67.5)
  line L240 (66.1596, 67.5) -> (66.1596, 62.5)
  line L241 (66.1596, 62.5) -> (71.0596, 62.5)
  line L242 (71.0596, 62.5) -> (71.0596, 60)
  line L243 (71.0596, 60) -> (76.4596, 60)
  line L244 (76.4596, 60) -> (76.4596, 62.5)
  line L245 (76.4596, 62.5) -> (81.0596, 62.5)
  line L246 (81.0596, 62.5) -> (81.0596, 60)
  line L247 (81.0596, 60) -> (86.4596, 60)
  line L248 (86.4596, 60) -> (86.4596, 62.5)
  line L249 (86.4596, 62.5) -> (91.0596, 62.5)
  line L250 (91.0596, 62.5) -> (91.0596, 60)
  line L251 (91.0596, 60) -> (96.4596, 60)
  line L252 (96.4596, 60) -> (96.4596, 62.5)
  line L253 (96.4596, 62.5) -> (101.0596, 62.5)
  line L254 (101.0596, 62.5) -> (101.0596, 60)
  line L255 (101.0596, 60) -> (106.4596, 60)
  line L256 (106.4596, 60) -> (106.4596, 62.5)
  line L257 (106.4596, 62.5) -> (116.1596, 62.5)
  line L258 (116.1596, 62.5) -> (116.1596, 67.5)
  line L259 (116.1596, 67.5) -> (113.1596, 67.5)
  line L260 (113.1596, 67.5) -> (113.1596, 72.5)
  line L261 (113.1596, 72.5) -> (116.1596, 72.5)
  line L262 (116.1596, 72.5) -> (116.1596, 77.5)
  line L263 (116.1596, 77.5) -> (113.1596, 77.5)
  line L264 (113.1596, 77.5) -> (113.1596, 82.5)
  line L265 (113.1596, 82.5) -> (116.1596, 82.5)
  line L266 (116.1596, 82.5) -> (116.1596, 87.5)
  line L267 (116.1596, 87.5) -> (113.1596, 87.5)
  line L268 (113.1596, 87.5) -> (113.1596, 92.5)
  line L269 (113.1596, 92.5) -> (116.1596, 92.5)
  line L270 (116.1596, 92.5) -> (116.1596, 97.5)
  line L271 (116.1596, 97.5) -> (113.1596, 97.5)
  line L272 (113.1596, 97.5) -> (113.1596, 102.5)
  line L273 (113.1596, 102.5) -> (116.1596, 102.5)
  line L274 (116.1596, 102.5) -> (116.1596, 107.5)
  line L275 (116.1596, 107.5) -> (66.1596, 107.5)
  line L276 (66.1596, 107.5) -> (66.1596, 102.5)
  line L277 (66.1596, 102.5) -> (68.1596, 102.5)
  line L278 (68.1596, 102.5) -> (68.1596, 97.5)
  line L279 (68.1596, 97.5) -> (66.1596, 97.5)
  line L280 (101.4074, 34.4317) -> (102.5829, 36.0497)
  arc A50 (105.5221, 33.1106) -> (102.5829, 36.0497) centre (94.774, 25.3016) ccw
  line L281 (105.5221, 33.1106) -> (103.9041, 31.935)
  arc A51 (103.9041, 31.935) -> (101.4074, 34.4317) centre (94.774, 25.3016) ccw
  line L282 (105.507, 21.8143) -> (107.4091, 21.1962)
  arc A52 (105.5221, 17.4927) -> (107.4091, 21.1962) centre (94.774, 25.3016) ccw
  line L283 (105.5221, 17.4927) -> (103.9041, 18.6683)
  arc A53 (103.9041, 18.6683) -> (105.507, 21.8143) centre (94.774, 25.3016) ccw
  arc A54 (90.6686, 12.6665) -> (94.774, 12.0163) centre (94.774, 25.3016) ccw
  line L284 (90.6686, 12.6665) -> (91.2866, 14.5686)
  arc A55 (91.2866, 14.5686) -> (94.774, 14.0163) centre (94.774, 25.3016) ccw
  line L285 (94.774, 14.0163) -> (94.774, 12.0163)
  line L286 (84.041, 21.8143) -> (82.1389, 21.1962)
  arc A56 (81.4886, 25.3016) -> (82.1389, 21.1962) centre (94.774, 25.3016) ccw
  line L287 (81.4886, 25.3016) -> (83.4886, 25.3016)
  arc A57 (83.4886, 25.3016) -> (84.041, 21.8143) centre (94.774, 25.3016) ccw
  line L288 (88.1406, 34.4317) -> (86.9651, 36.0497)
  arc A58 (90.6686, 37.9368) -> (86.9651, 36.0497) centre (94.774, 25.3016) ccw
  line L289 (90.6686, 37.9368) -> (91.2866, 36.0347)
  arc A59 (91.2866, 36.0347) -> (88.1406, 34.4317) centre (94.774, 25.3016) ccw
  line L290 (84.041, 28.789) -> (82.1389, 29.407)
  arc A60 (84.0259, 33.1106) -> (82.1389, 29.407) centre (94.774, 25.3016) ccw
  line L291 (84.0259, 33.1106) -> (85.644, 31.935)
  arc A61 (85.644, 31.935) -> (84.041, 28.789) centre (94.774, 25.3016) ccw
  line L292 (88.1406, 16.1716) -> (86.9651, 14.5536)
  arc A62 (84.0259, 17.4927) -> (86.9651, 14.5536) centre (94.774, 25.3016) ccw
  line L293 (84.0259, 17.4927) -> (85.644, 18.6683)
  arc A63 (85.644, 18.6683) -> (88.1406, 16.1716) centre (94.774, 25.3016) ccw
  line L294 (101.4074, 16.1716) -> (102.5829, 14.5536)
  arc A64 (98.8794, 12.6665) -> (102.5829, 14.5536) centre (94.774, 25.3016) ccw
  line L295 (98.8794, 12.6665) -> (98.2614, 14.5686)
  arc A65 (98.2614, 14.5686) -> (101.4074, 16.1716) centre (94.774, 25.3016) ccw
  line L296 (105.507, 28.789) -> (107.4091, 29.407)
  arc A66 (108.0594, 25.3016) -> (107.4091, 29.407) centre (94.774, 25.3016) ccw
  line L297 (108.0594, 25.3016) -> (106.0594, 25.3016)
  arc A67 (106.0594, 25.3016) -> (105.507, 28.789) centre (94.774, 25.3016) ccw
  arc A68 (98.8794, 37.9368) -> (94.774, 38.587) centre (94.774, 25.3016) ccw
  line L298 (98.8794, 37.9368) -> (98.2614, 36.0347)
  arc A69 (98.2614, 36.0347) -> (94.774, 36.587) centre (94.774, 25.3016) ccw
  line L299 (94.774, 36.587) -> (94.774, 38.587)
  line L300 (103.7585, 37.6678) -> (104.9341, 39.2858)
  arc A70 (108.7582, 35.4617) -> (104.9341, 39.2858) centre (94.774, 25.3016) ccw
  line L301 (108.7582, 35.4617) -> (107.1401, 34.2862)
  arc A71 (107.1401, 34.2862) -> (103.7585, 37.6678) centre (94.774, 25.3016) ccw
  line L302 (109.3112, 20.5782) -> (111.2134, 19.9602)
  arc A72 (108.7582, 15.1416) -> (111.2134, 19.9602) centre (94.774, 25.3016) ccw
  line L303 (108.7582, 15.1416) -> (107.1401, 16.3171)
  arc A73 (107.1401, 16.3171) -> (109.3112, 20.5782) centre (94.774, 25.3016) ccw
  arc A74 (89.4325, 8.8623) -> (94.774, 8.0163) centre (94.774, 25.3016) ccw
  line L304 (89.4325, 8.8623) -> (90.0506, 10.7644)
  arc A75 (90.0506, 10.7644) -> (94.774, 10.0163) centre (94.774, 25.3016) ccw
  line L305 (94.774, 10.0163) -> (94.774, 8.0163)
  line L306 (80.2368, 20.5782) -> (78.3347, 19.9602)
  arc A76 (77.4886, 25.3016) -> (78.3347, 19.9602) centre (94.774, 25.3016) ccw
  line L307 (77.4886, 25.3016) -> (79.4886, 25.3016)
  arc A77 (79.4886, 25.3016) -> (80.2368, 20.5782) centre (94.774, 25.3016) ccw
  arc A78 (97.6433, 34.1325) -> (94.774, 34.587) centre (94.774, 25.3016) ccw
  line L308 (97.6433, 34.1325) -> (94.774, 25.3016)
  line L309 (94.774, 25.3016) -> (100.2318, 32.8137)
  arc A79 (102.286, 30.7594) -> (100.2318, 32.8137) centre (94.774, 25.3016) ccw
  line L310 (102.286, 30.7594) -> (94.774, 25.3016)
  line L311 (94.774, 25.3016) -> (103.6049, 28.171)
  arc A80 (104.0594, 25.3016) -> (103.6049, 28.171) centre (94.774, 25.3016) ccw
  line L312 (104.0594, 25.3016) -> (94.774, 25.3016)
  line L313 (94.774, 25.3016) -> (103.6049, 22.4323)
  arc A81 (102.286, 19.8438) -> (103.6049, 22.4323) centre (94.774, 25.3016) ccw
  line L314 (102.286, 19.8438) -> (94.774, 25.3016)
  line L315 (94.774, 25.3016) -> (100.2318, 17.7896)
  arc A82 (97.6433, 16.4707) -> (100.2318, 17.7896) centre (94.774, 25.3016) ccw
  line L316 (97.6433, 16.4707) -> (94.774, 25.3016)
  line L317 (94.774, 25.3016) -> (94.774, 16.0163)
  arc A83 (91.9047, 16.4707) -> (94.774, 16.0163) centre (94.774, 25.3016) ccw
  line L318 (91.9047, 16.4707) -> (94.774, 25.3016)
  line L319 (94.774, 25.3016) -> (89.3162, 17.7896)
  arc A84 (87.262, 19.8438) -> (89.3162, 17.7896) centre (94.774, 25.3016) ccw
  line L320 (87.262, 19.8438) -> (94.774, 25.3016)
  line L321 (94.774, 25.3016) -> (85.9431, 22.4323)
  arc A85 (85.4886, 25.3016) -> (85.9431, 22.4323) centre (94.774, 25.3016) ccw
  line L322 (85.4886, 25.3016) -> (94.774, 25.3016)
  line L323 (94.774, 25.3016) -> (85.9431, 28.171)
  arc A86 (87.262, 30.7594) -> (85.9431, 28.171) centre (94.774, 25.3016) ccw
  line L324 (87.262, 30.7594) -> (94.774, 25.3016)
  line L325 (94.774, 25.3016) -> (89.3162, 32.8137)
  arc A87 (91.9047, 34.1325) -> (89.3162, 32.8137) centre (94.774, 25.3016) ccw
  line L326 (91.9047, 34.1325) -> (94.774, 25.3016)
  line L327 (94.774, 25.3016) -> (94.774, 34.587)
  line L328 (85.7895, 37.6678) -> (84.6139, 39.2858)
  arc A88 (89.4325, 41.741) -> (84.6139, 39.2858) centre (94.774, 25.3016) ccw
  line L329 (89.4325, 41.741) -> (90.0506, 39.8389)
  arc A89 (90.0506, 39.8389) -> (85.7895, 37.6678) centre (94.774, 25.3016) ccw
  line L330 (80.2368, 30.0251) -> (78.3347, 30.6431)
  arc A90 (80.7899, 35.4617) -> (78.3347, 30.6431) centre (94.774, 25.3016) ccw
  line L331 (80.7899, 35.4617) -> (82.4079, 34.2862)
  arc A91 (82.4079, 34.2862) -> (80.2368, 30.0251) centre (94.774, 25.3016) ccw
  line L332 (85.7895, 12.9355) -> (84.6139, 11.3175)
  arc A92 (80.7899, 15.1416) -> (84.6139, 11.3175) centre (94.774, 25.3016) ccw
  line L333 (80.7899, 15.1416) -> (82.4079, 16.3171)
  arc A93 (82.4079, 16.3171) -> (85.7895, 12.9355) centre (94.774, 25.3016) ccw
  line L334 (103.7585, 12.9355) -> (104.9341, 11.3175)
  arc A94 (100.1155, 8.8623) -> (104.9341, 11.3175) centre (94.774, 25.3016) ccw
  line L335 (100.1155, 8.8623) -> (99.4974, 10.7644)
  arc A95 (99.4974, 10.7644) -> (103.7585, 12.9355) centre (94.774, 25.3016) ccw
  line L336 (109.3112, 30.0251) -> (111.2134, 30.6431)
  arc A96 (112.0594, 25.3016) -> (111.2134, 30.6431) centre (94.774, 25.3016) ccw
  line L337 (112.0594, 25.3016) -> (110.0594, 25.3016)
  arc A97 (110.0594, 25.3016) -> (109.3112, 30.0251) centre (94.774, 25.3016) ccw
  arc A98 (100.1155, 41.741) -> (94.774, 42.587) centre (94.774, 25.3016) ccw
  line L338 (100.1155, 41.741) -> (99.4974, 39.8389)
  arc A99 (99.4974, 39.8389) -> (94.774, 40.587) centre (94.774, 25.3016) ccw
  line L339 (94.774, 40.587) -> (94.774, 42.587)
  line L340 (117.5, 0) -> (117.5, 7.3)
  line L341 (117.5, 7.3) -> (120, 7.3)
  line L342 (120, 7.3) -> (120, 12.7)
  line L343 (120, 12.7) -> (117.5, 12.7)
  line L344 (117.5, 12.7) -> (117.5, 17.3)
  line L345 (117.5, 17.3) -> (120, 17.3)
  line L346 (120, 17.3) -> (120, 22.7)
  line L347 (120, 22.7) -> (117.5, 22.7)
  line L348 (117.5, 22.7) -> (117.5, 27.3)
  line L349 (117.5, 27.3) -> (120, 27.3)
  line L350 (120, 27.3) -> (120, 32.7)
  line L351 (120, 32.7) -> (117.5, 32.7)
  line L352 (117.5, 32.7) -> (117.5, 37.3)
  line L353 (117.5, 37.3) -> (120, 37.3)
  line L354 (120, 37.3) -> (120, 42.7)
  line L355 (120, 42.7) -> (117.5, 42.7)
  line L356 (117.5, 42.7) -> (117.5, 47.5)
  line L357 (117.5, 47.5) -> (72.5, 47.5)
  line L358 (72.5, 47.5) -> (72.5, 42.7)
  line L359 (72.5, 42.7) -> (70, 42.7)
  line L360 (70, 42.7) -> (70, 37.3)
  line L361 (70, 37.3) -> (72.5, 37.3)
  line L362 (72.5, 37.3) -> (72.5, 32.7)
  line L363 (72.5, 32.7) -> (70, 32.7)
  line L364 (70, 32.7) -> (70, 27.3)
  line L365 (70, 27.3) -> (72.5, 27.3)
  line L366 (72.5, 27.3) -> (72.5, 22.7)
  line L367 (72.5, 22.7) -> (70, 22.7)
  line L368 (70, 22.7) -> (70, 17.3)
  line L369 (70, 17.3) -> (72.5, 17.3)
  line L370 (72.5, 17.3) -> (72.5, 12.7)
  line L371 (72.5, 12.7) -> (70, 12.7)
  line L372 (70, 12.7) -> (70, 7.3)
  line L373 (70, 7.3) -> (72.5, 7.3)
  line L374 (72.5, 7.3) -> (72.5, 0)
  line L375 (72.5, 0) -> (77.5, 0)
  line L376 (77.5, 0) -> (77.5, 3)
  line L377 (77.5, 3) -> (82.5, 3)
  line L378 (82.5, 3) -> (82.5, 0)
  line L379 (82.5, 0) -> (87.5, 0)
  line L380 (87.5, 0) -> (87.5, 3)
  line L381 (87.5, 3) -> (92.5, 3)
  line L382 (92.5, 3) -> (92.5, 0)
  line L383 (92.5, 0) -> (97.5, 0)
  line L384 (97.5, 0) -> (97.5, 3)
  line L385 (97.5, 3) -> (102.5, 3)
  line L386 (102.5, 3) -> (102.5, 0)
  line L387 (102.5, 0) -> (107.5, 0)
  line L388 (107.5, 0) -> (107.5, 3)
  line L389 (107.5, 3) -> (112.5, 3)
  line L390 (112.5, 3) -> (112.5, 0)
  line L391 (112.5, 0) -> (117.5, 0)
  spline S0 degree 3 poles (28.7467, 4.3909) (28.6234, 4.4633) (28.3825, 4.6049) (28.1964, 4.8131) (28.1055, 4.9148) knots 0 0 0 0 0.042587 0.083249 0.083249 0.083249 0.083249
  line L392 (28.1055, 4.9148) -> (28.1055, 2.0935)
  line L393 (28.1055, 2.0935) -> (27.1232, 2.0935)
  line L394 (27.1232, 2.0935) -> (27.1232, 10.1099)
  line L395 (27.1232, 10.1099) -> (28.0181, 10.1099)
  line L396 (28.0181, 10.1099) -> (28.0181, 9.3568)
  spline S1 degree 3 poles (28.0181, 9.3568) (28.1237, 9.4931) (28.3257, 9.7536) (28.6015, 9.9339) (28.733, 10.0199) knots 0 0 0 0 0.051297 0.098108 0.098108 0.098108 0.098108
  spline S2 degree 3 poles (28.733, 10.0199) (28.8777, 10.0843) (29.1848, 10.2209) (29.5211, 10.234) (29.6989, 10.2409) knots 0 0 0 0 0.04708 0.099894 0.099894 0.099894 0.099894
  spline S3 degree 3 poles (29.6989, 10.2409) (29.9369, 10.2264) (30.4026, 10.198) (30.8096, 9.9703) (31.0086, 9.8589) knots 0 0 0 0 0.0705 0.138 0.138 0.138 0.138
  spline S4 degree 3 poles (31.0086, 9.8589) (31.1873, 9.7156) (31.5543, 9.4215) (31.7599, 8.9982) (31.8653, 8.7811) knots 0 0 0 0 0.06782 0.139223 0.139223 0.139223 0.139223
  spline S5 degree 3 poles (31.8653, 8.7811) (31.9497, 8.5404) (32.1226, 8.0467) (32.1438, 7.5238) (32.1546, 7.2559) knots 0 0 0 0 0.076078 0.156009 0.156009 0.156009 0.156009
  spline S6 degree 3 poles (32.1546, 7.2559) (32.1432, 6.9711) (32.1211, 6.4201) (31.9284, 5.9037) (31.8353, 5.6542) knots 0 0 0 0 0.084892 0.164238 0.164238 0.164238 0.164238
  spline S7 degree 3 poles (31.8353, 5.6542) (31.7193, 5.4322) (31.4922, 4.9981) (31.0995, 4.7057) (30.9076, 4.5628) knots 0 0 0 0 0.074084 0.144891 0.144891 0.144891 0.144891
  spline S8 degree 3 poles (30.9076, 4.5628) (30.7042, 4.4522) (30.3044, 4.2348) (29.8508, 4.2004) (29.628, 4.1836) knots 0 0 0 0 0.068591 0.134825 0.134825 0.134825 0.134825
  spline S9 degree 3 poles (29.628, 4.1836) (29.4704, 4.1912) (29.1636, 4.2061) (28.8831, 4.3305) (28.7467, 4.3909) knots 0 0 0 0 0.046877 0.091235 0.091235 0.091235 0.091235
  line L397 (21.8599, 16.8002) -> (19.5461, 23.6106)
  line L398 (19.5461, 23.6106) -> (19.5461, 16.8002)
  line L399 (19.5461, 16.8002) -> (18.5256, 16.8002)
  line L400 (18.5256, 16.8002) -> (18.5256, 24.8002)
  line L401 (18.5256, 24.8002) -> (20.1191, 24.8002)
  line L402 (20.1191, 24.8002) -> (22.0127, 19.1358)
  spline S10 degree 3 poles (22.0127, 19.1358) (22.0889, 18.9055) (22.2192, 18.5117) (22.3432, 18.1159) (22.3947, 17.9516) knots 0 0 0 0 0.072781 0.124428 0.124428 0.124428 0.124428
  spline S11 degree 3 poles (22.3947, 17.9516) (22.4524, 18.1314) (22.5902, 18.5603) (22.7358, 18.9865) (22.8203, 19.234) knots 0 0 0 0 0.056647 0.135122 0.135122 0.135122 0.135122
  line L403 (22.8203, 19.234) -> (24.7357, 24.8002)
  line L404 (24.7357, 24.8002) -> (26.16, 24.8002)
  line L405 (26.16, 24.8002) -> (26.16, 16.8002)
  line L406 (26.16, 16.8002) -> (25.1396, 16.8002)
  line L407 (25.1396, 16.8002) -> (25.1396, 23.496)
  line L408 (25.1396, 23.496) -> (22.8149, 16.8002)
  line L409 (22.8149, 16.8002) -> (21.8599, 16.8002)
  spline S12 degree 3 poles (21.8271, 30.4701) (22.0001, 30.322) (22.3494, 30.0232) (22.8074, 29.9829) (23.0386, 29.9626) knots 0 0 0 0 0.066533 0.134307 0.134307 0.134307 0.134307
  spline S13 degree 3 poles (23.0386, 29.9626) (23.2097, 29.9727) (23.5407, 29.9922) (23.824, 30.1636) (23.9608, 30.2463) knots 0 0 0 0 0.050568 0.097791 0.097791 0.097791 0.097791
  spline S14 degree 3 poles (23.9608, 30.2463) (24.0842, 30.3628) (24.3544, 30.6178) (24.4919, 30.964) (24.5666, 31.1522) knots 0 0 0 0 0.050293 0.110147 0.110147 0.110147 0.110147
  line L410 (24.5666, 31.1522) -> (25.5816, 31.0267)
  spline S15 degree 3 poles (25.5816, 31.0267) (25.4883, 30.7497) (25.3079, 30.2138) (24.8927, 29.831) (24.6921, 29.646) knots 0 0 0 0 0.086093 0.166606 0.166606 0.166606 0.166606
  spline S16 degree 3 poles (24.6921, 29.646) (24.4518, 29.5029) (23.9418, 29.1991) (23.3475, 29.1702) (23.0332, 29.1549) knots 0 0 0 0 0.08261 0.175377 0.175377 0.175377 0.175377
  spline S17 degree 3 poles (23.0332, 29.1549) (22.6376, 29.1811) (21.8812, 29.2313) (21.296, 29.7097) (21.0168, 29.938) knots 0 0 0 0 0.115653 0.221163 0.221163 0.221163 0.221163
  spline S18 degree 3 poles (21.0168, 29.938) (20.7998, 30.2406) (20.3312, 30.8944) (20.2926, 31.7011) (20.2719, 32.1345) knots 0 0 0 0 0.109405 0.236358 0.236358 0.236358 0.236358
  spline S19 degree 3 poles (20.2719, 32.1345) (20.2923, 32.5821) (20.3302, 33.4131) (20.8057, 34.0916) (21.025, 34.4046) knots 0 0 0 0 0.131235 0.243597 0.243597 0.243597 0.243597
  spline S20 degree 3 poles (21.025, 34.4046) (21.2992, 34.6401) (21.8609, 35.1226) (22.6002, 35.1819) (22.9786, 35.2122) knots 0 0 0 0 0.105595 0.216319 0.216319 0.216319 0.216319
  spline S21 degree 3 poles (22.9786, 35.2122) (23.3457, 35.182) (24.065, 35.1229) (24.6105, 34.6517) (24.8776, 34.4209) knots 0 0 0 0 0.10743 0.210533 0.210533 0.210533 0.210533
  spline S22 degree 3 poles (24.8776, 34.4209) (25.0922, 34.1141) (25.5575, 33.4484) (25.5944, 32.6336) (25.6143, 32.1945) knots 0 0 0 0 0.110094 0.238839 0.238839 0.238839 0.238839
  spline S23 degree 3 poles (25.6143, 32.1945) (25.614, 32.1581) (25.6131, 32.0708) (25.6104, 31.9835) (25.6089, 31.9325) knots 0 0 0 0 0.010915 0.0262 0.0262 0.0262 0.0262
  line L411 (25.6089, 31.9325) -> (21.2869, 31.9325)
  spline S24 degree 3 poles (21.2869, 31.9325) (21.3153, 31.6416) (21.3677, 31.1047) (21.6828, 30.6694) (21.8271, 30.4701) knots 0 0 0 0 0.08586 0.158415 0.158415 0.158415 0.158415
  spline S25 degree 3 poles (28.9704, 17.9844) (29.1434, 17.8364) (29.4926, 17.5376) (29.9507, 17.4972) (30.1819, 17.4769) knots 0 0 0 0 0.066533 0.134307 0.134307 0.134307 0.134307
  spline S26 degree 3 poles (30.1819, 17.4769) (30.353, 17.487) (30.684, 17.5066) (30.9673, 17.6779) (31.1041, 17.7606) knots 0 0 0 0 0.050568 0.097792 0.097792 0.097792 0.097792
  spline S27 degree 3 poles (31.1041, 17.7606) (31.2275, 17.8771) (31.4976, 18.1321) (31.6351, 18.4784) (31.7098, 18.6665) knots 0 0 0 0 0.050293 0.110147 0.110147 0.110147 0.110147
  line L412 (31.7098, 18.6665) -> (32.7248, 18.541)